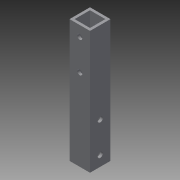
# Autodesk Inventor part: SuperStructureSupport
Saved by Autodesk Inventor 2013 (Build 170138000, 138)
## iProperties
Created: 2014-01-18
Part Number: SuperStructureSupport
Material: Generic
Document SubType Name: Modeling
Designer: 215152
Density: 1 g/cm^3
Author: 215152
Autodesk Inventor part; units mm, degrees
ref_plane "YZ Plane" through (0, 0, 0) normal (1, 0, 0) x (0, 1, 0)
ref_plane "XZ Plane" through (0, 0, 0) normal (0, 1, 0) x (-1, 0, 0)
ref_plane "XY Plane" through (0, 0, 0) normal (0, 0, 1) x (1, 0, 0)
sketch "Sketch1" plane through (0, 0, 0) normal (0, 1, 0) x (-1, 0, 0)
  line L0 (-12.7, -12.7) -> (12.7, -12.7)
  line L1 (12.7, -12.7) -> (12.7, 12.7)
  line L2 (12.7, 12.7) -> (-12.7, 12.7)
  line L3 (-12.7, 12.7) -> (-12.7, -12.7)
  line L4 (-12.7, -12.7) -> (12.7, 12.7) construction
  line L5 (12.7, -12.7) -> (-12.7, 12.7) construction
  line L6 (-9.525, -9.525) -> (9.525, -9.525)
  line L7 (9.525, -9.525) -> (9.525, 9.525)
  line L8 (9.525, 9.525) -> (-9.525, 9.525)
  line L9 (-9.525, 9.525) -> (-9.525, -9.525)
  line L10 (-9.525, -9.525) -> (9.525, 9.525) construction
  line L11 (9.525, -9.525) -> (-9.525, 9.525) construction
  point P0 (0, 0)
  dimension "d0" = 25.4
  dimension "d1" = 25.4
  dimension "d2" = 19.05
  dimension "d3" = 19.05
  constraints: 24 end point, 4 midpoint, 4 parallel, 2 horizontal, 2 perpendicular
  measures "d0" distance of L2.end L1.end
  measures "d1" distance of L1.end L0.end
  measures "d2" distance of L8.end L7.end
  measures "d3" distance of L7.end L6.end
extrude "Extrusion1" add sketch "Sketch1" along normal blind 152.4
sketch "Sketch2" plane through (-12.7, 0, 12.7) normal (0, 0, 1) x (1, 0, 0)
  line L0 (0, 152.4) -> (25.4, 152.4) projected
  line L1 (0, 0) -> (0, 152.4) projected
  line L2 (12.7, 152.4) -> (12.7, 139.7)
  line L3 (12.7, 139.7) -> (12.7, 101.6)
  circle A0 centre (12.7, 139.7) radius 3.175
  circle A1 centre (12.7, 101.6) radius 3.175
  point P0 (12.7, 0)
  dimension "d6" = 12.7
  dimension "d7" = 38.1
  dimension "d8" = 180
  dimension "d9" = 6.35
  dimension "d10" = 6.35
  constraints: 4 end point, 2 centre point, 2 coincident, 1 collinear, 1 midpoint, 1 parallel
  measures "d6" distance of L2.start L2.end
  measures "d7" distance of L2.end L3.end
  measures "d8" angle of L3 L2
  measures "d9" diameter of A0
  measures "d10" diameter of A1
extrude "Extrusion2" cut sketch "Sketch2" against normal blind 25.4
sketch "Sketch3" plane through (12.7, 0, 12.7) normal (1, 0, 0) x (0, 0, -1)
  line L0 (0, 0) -> (0, 152.4) projected
  line L1 (12.7, 0) -> (12.7, 12.7)
  line L2 (12.7, 0) -> (25.4, 0) construction
  line L3 (12.7, 12.7) -> (12.7, 50.8)
  line L4 (12.7, 12.7) -> (50.8, 12.7) construction
  circle A0 centre (12.7, 50.8) radius 3.175
  circle A1 centre (12.7, 12.7) radius 3.175
  dimension "d13" = 12.7
  dimension "d14" = 90
  dimension "d15" = 38.1
  dimension "d16" = 90
  dimension "d17" = 6.35
  dimension "d18" = 6.35
  constraints: 8 end point, 3 perpendicular, 2 centre point, 2 coincident, 2 horizontal, 1 parallel
  measures "d13" distance of L1.start L1.end
  measures "d14" angle of L2 L1
  measures "d15" distance of L1.end L3.end
  measures "d16" angle of L4 L3
  measures "d17" diameter of A0
  measures "d18" diameter of A1
extrude "Extrusion3" cut sketch "Sketch3" against normal blind 25.4
body "Solid1"
